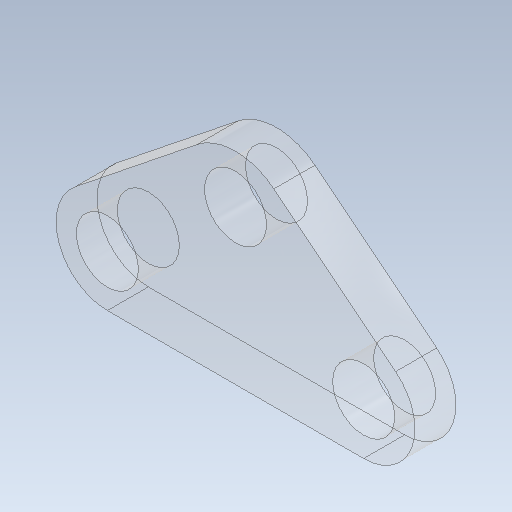
# Autodesk Inventor part: アーム詰め物
Saved by Autodesk Inventor 2020.4 (Build 244396000, 396)
## iProperties
Created: 2021-05-02
Part Number: アーム詰め物
Material: ポリカーボネート、クリア
Document SubType Name: Modeling
Designer: happy
Density: 1.2 g/cm^3
Appearance: ポリカーボネート - クリア
Mass: 1.92479 g
Surface Area: 13.828 cm^2
Volume: 1.60399 cm^3
Author: happy
Autodesk Inventor part; units mm, degrees
ref_plane "YZ Plane" through (0, 0, 0) normal (1, 0, 0) x (0, 1, 0)
ref_plane "XZ Plane" through (0, 0, 0) normal (0, 1, 0) x (-1, 0, 0)
ref_plane "XY Plane" through (0, 0, 0) normal (0, 0, 1) x (1, 0, 0)
sketch "スケッチ1" plane through (0, 0, 0) normal (0, 0, 1) x (1, 0, 0)
  line L0 (92.493, 12) -> (30.0122, 12)
  arc A0 (30.0122, 12) -> (23.3428, 9.9759) centre (30.0122, 0) ccw
  arc A1 (6.6694, 9.9759) -> (23.3428, 9.9759) centre (15.0061, 22.4459) ccw
  arc A2 (6.6694, 9.9759) -> (0, -12) centre (0, 0) ccw
  line L1 (0, -12) -> (30, -12)
  arc A3 (30, -12) -> (30, -12) centre (30, 0) ccw construction
  line L2 (30, -12) -> (92.493, -12)
  line L3 (92.493, -12) -> (92.493, 12)
  circle A4 centre (30, 0) radius 9.025 construction
  circle A5 centre (0, 0) radius 1.5
  circle A6 centre (16, 0) radius 1.25
  circle A7 centre (48, -5) radius 3.025
  circle A8 centre (73, -5) radius 3.025
  circle A9 centre (60.5, 5) radius 3.025
  line L4 (48, -5) -> (73, -5) construction
  line L5 (92.493, 12) -> (30.0122, 12)
  line L6 (59.7539, 12) -> (92.493, -14.1913)
  line L7 (92.493, -12) -> (92.493, 12)
  line L8 (60.5, 5) -> (73, -5) construction
  line L9 (60.5, 5) -> (60.5, -5) construction
  line L10 (61.2461, 12) -> (28.507, -14.1913)
  arc A10 (44.8765, -1.0957) -> (48, -10) centre (48, -5) ccw
  arc A11 (73, -10) -> (76.1235, -1.0957) centre (73, -5) ccw
  line L11 (48, -10) -> (73, -10)
  point P0 (60.5, 0)
  point P1 (61.3547, 12)
  point P2 (91.3547, -12)
  point P3 (59.6453, 12)
  point P4 (29.6453, -12)
  point P5 (89.7539, -12)
  point P6 (60.5, 11.4031)
  point P7 (31.2461, -12)
  dimension "d0" = 6.05
  dimension "d1" = 6.05
  dimension "d2" = 6.05
  dimension "d3" = 25
  dimension "d4" = 10
  dimension "d5" = 18
  dimension "d6" = 5
  constraints: 24 end point, 12 centre point, 12 point on circle, 4 midpoint, 3 tangent, 2 coincident, 2 horizontal, 2 parallel, 2 point on line, 2 symmetric about line, 1 horizontal alignment, 1 vertical, 1 vertical alignment, 10 other
  measures "d0" diameter of A7
  measures "d1" diameter of A8
  measures "d2" diameter of A9
  measures "d3" distance of L4.end L4.start
  measures "d4" vertical distance of L8.start L4.start
  measures "d5" horizontal distance of A4.centre L4.start
  measures "d6" distance between parallel lines of L6 L8
extrude "押し出し1" add sketch "スケッチ1" along normal blind 4 contours L6 A11 L11 A10 L10
fillet "フィレット3" radius 6 1 edges at (60.5, 11.4031, 2)
